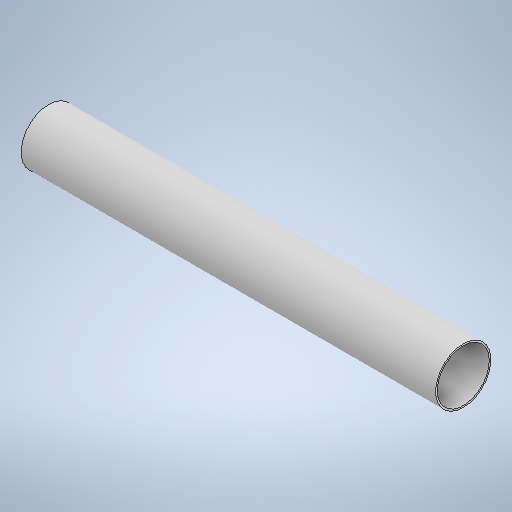
# Autodesk Inventor part: Peça5
Saved by Autodesk Inventor 2025.2 (Build 292293000, 293)
## iProperties
Created: 2025-03-25
Part Number: Peça5
Material: Genérico
Document SubType Name: Modeling
Designer: Formação
Density: 1 g/cm^3
Appearance: Padrão
Author: Formação
Autodesk Inventor part; units mm, degrees
ref_plane "YZ Plane" through (0, 0, 0) normal (1, 0, 0) x (0, 1, 0)
ref_plane "XZ Plane" through (0, 0, 0) normal (0, 1, 0) x (-1, 0, 0)
ref_plane "XY Plane" through (0, 0, 0) normal (0, 0, 1) x (1, 0, 0)
sketch "Esboço1" plane through (0, 0, 0) normal (0, 0, 1) x (1, 0, 0)
  line L0 (-375, 50) -> (375, 50)
  line L1 (375, 50) -> (375, 47)
  line L2 (375, 47) -> (-375, 47)
  line L3 (-375, 47) -> (-375, 50)
  line L4 (-375, 50) -> (375, 47) construction
  line L5 (375, 50) -> (-375, 47) construction
  line L6 (38, 2) -> (157.733, 10)
  line L7 (-525, 0) -> (525, 0) projected
  point P0 (0, 0)
  point P1 (0, 48.5)
  dimension "d0" = 750
  dimension "d1" = 50
  dimension "d2" = 3
  dimension "d3" = 120
  constraints: 14 end point, 2 midpoint, 2 parallel, 1 horizontal, 1 perpendicular, 1 vertical alignment
  measures "d0" distance of L1.end L2.end
  measures "d1" distance from line of point (0, 0) L0
  measures "d2" distance of L2.end L0.start
  measures "d3" distance of L6.start L6.end
revolve "Revolução1" add sketch "Esboço1" angle 360 about axis through (-10, 0, 0) along (1, 0, 0)
